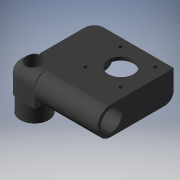
# Autodesk Inventor part: zmotormount
Saved by Autodesk Inventor 2019.1 (Build 231200000, 200)
## iProperties
Created: 2019-08-11
Part Number: zmotormount
Material: Generic
Document SubType Name: Modeling
Designer: rob
Density: 1 g/cm^3
Appearance: Default
Author: rob
## iProperties of the stored document zmotormount_3DPrint.ipt
Created: 2019-08-11
Part Number: zmotormount_3DPrint
Material: Generic
Document SubType Name: Modeling
Designer: rob
Density: 1 g/cm^3
Appearance: Default
Author: rob
Autodesk Inventor part; units mm, degrees
ref_plane "YZ Plane" through (0, 0, 0) normal (1, 0, 0) x (0, 1, 0)
ref_plane "XZ Plane" through (0, 0, 0) normal (0, 1, 0) x (-1, 0, 0)
ref_plane "XY Plane" through (0, 0, 0) normal (0, 0, 1) x (1, 0, 0)
sketch "Sketch1" plane through (0, 0, 0) normal (0, 1, 0) x (-1, 0, 0)
  circle A0 centre (0, 0) radius 9.125
  circle A1 centre (0, 0) radius 12.5
  dimension "d0" = 18.25
  dimension "d1" = 25
  constraints: 2 centre point, 2 coincident
  measures "d0" diameter of A0
  measures "d1" diameter of A1
extrude "Extrusion1" add sketch "Sketch1" along normal blind 15
sketch "Sketch2" plane through (0, 15, 0) normal (0, 1, 0) x (1, 0, 0)
  line L0 (-12.5, -12.5) -> (12.5, -12.5)
  line L1 (12.5, -12.5) -> (12.5, 12.5)
  line L2 (12.5, 12.5) -> (-12.5, 12.5)
  line L3 (-12.5, 12.5) -> (-12.5, -12.5)
  point P0 (0, 0)
  constraints: 8 end point, 2 parallel, 1 horizontal, 1 perpendicular
extrude "Extrusion2" add sketch "Sketch2" along normal blind 25
sketch "Sketch3" plane through (12.5, 15, 12.5) normal (1, 0, 0) x (0, 0, -1)
  circle A0 centre (12.5, 12.5) radius 12.5
  circle A1 centre (12.5, 12.5) radius 9.125
  point P0 (12.5, -15)
  dimension "d6" = 25
  dimension "d7" = 18.25
  constraints: 2 centre point, 1 coincident
  measures "d6" diameter of A0
  measures "d7" diameter of A1
extrude "Extrusion3" add sketch "Sketch3" along normal blind 53.5
fillet "Fillet1" radius 10 5 edges at (0, 40, -12.5) (-12.5, 40, 0) (0, 40, 12.5) (-12.5, 27.5, 12.5) (-12.5, 27.5, -12.5)
sketch "Sketch4" plane through (0, 40, 0) normal (0, 1, 0) x (1, 0, 0)
  circle A0 centre (43.7484, 32.8534) radius 11.25
  circle A1 centre (43.7484, 32.8534) radius 2.75
  circle A2 centre (28.2484, 17.3534) radius 1.75
  circle A3 centre (28.2484, 48.3534) radius 1.75
  circle A4 centre (59.2484, 48.3534) radius 1.75
  circle A5 centre (59.2484, 17.3534) radius 1.75
  line L0 (-2.5, -2.5) -> (-2.5, 2.5) projected
  line L1 (-2.5, -2.5) -> (55.5607, -2.5)
  line L2 (66, -2.5) -> (66, 83.8642)
  line L3 (55.5607, 83.8642) -> (-2.5, 83.8642)
  line L4 (-2.5, 83.8642) -> (-2.5, -2.5)
  line L5 (-47.4497, 33) -> (137.0981, 33)
  line L6 (43.6, -25.832) -> (43.6, 75.2549)
  line L7 (55.5607, 83.8642) -> (66, 83.8642)
  line L8 (66, -2.5) -> (47.9455, -2.5)
  line L9 (66, -12.5) -> (66, 12.5) projected
  point P0 (0, 0)
  dimension "d13" = 22.5
  dimension "d14" = 5.5
  dimension "d15" = 3.5
  dimension "d16" = 15.5
  dimension "d20" = 360
  dimension "d37" = 33
  dimension "d43" = 43.6
  dimension "d44" = 0
  constraints: 16 end point, 6 centre point, 3 coincident, 3 horizontal, 2 parallel, 1 perpendicular, 1 point on line, 1 vertical, 10 other
  measures "d13" diameter of A0
  measures "d14" diameter of A1
  measures "d15" diameter of A2
  measures "d16" horizontal distance of A2.centre A0.centre
  measures "d37" distance from line of L5 point (0, 0)
  measures "d43" distance from line of L6 point (0, 0)
  measures "d44" distance between parallel lines of L9 L2
extrude "Extrusion4" add sketch "Sketch4" against normal blind 3 contours A0 L5 L2 L8 L1 L6 | A0 L5 L4 L3 L7 L2 | L6 L1 L0 L4 L5 A0
fillet "Fillet2" radius 40 1 edges at (-2.5, 38.5, -83.8642)
fillet "Fillet3" radius 10 1 edges at (66, 38.5, -83.8642)
sketch "Sketch5" plane through (66, 27.5, 0) normal (1, 0, 0) x (0, 0, -1)
  circle A0 centre (0, 0) radius 12.5
  line L0 (0, -12.5) -> (-12.5, -12.5) projected
  line L1 (0, -12.5) -> (73.8642, -12.5)
  line L2 (83.8642, 9.5) -> (83.8642, 12.5) projected
  line L3 (73.8642, -12.5) -> (73.8642, 12.5)
  line L4 (73.8642, 12.5) -> (0, 12.5)
  circle A1 centre (0, 0) radius 9.125
  line L5 (73.8642, 12.5) -> (73.8642, 9.5) projected
  point P0 (0, -27.5)
  dimension "d28" = 0
  dimension "d45" = 18.25
  constraints: 5 end point, 2 centre point, 2 tangent, 1 coincident, 1 collinear, 1 perpendicular, 1 point on circle, 1 point on line
  measures "d28" distance between parallel lines of L5 L3
  measures "d45" diameter of A1
extrude "Extrusion5" add sketch "Sketch5" along normal blind 2
fillet "Fillet5" radius 8 2 edges at (67, 15, -73.8642) (68, 27.5, -73.8642)
sketch "Sketch6" plane through (12.5, 15, 0) normal (1, 0, 0) x (0, 0, -1)
  line L0 (12.5, 15) -> (12.5, 0) projected
  line L1 (12.5, 0) -> (65.8642, 0)
  line L2 (0, 0) -> (65.8642, 0) projected
  line L3 (65.8642, 0) -> (65.8642, 22)
  line L4 (44.1034, 22) -> (21.6034, 22) projected
  line L5 (65.8642, 0) -> (12.5, 0)
  line L6 (12.5, 0) -> (12.5, 22)
  line L7 (12.5, 22) -> (65.8642, 22)
  line L8 (65.8642, 22) -> (65.8642, 0)
  point P0 (0, -15)
  point P1 (12.5, 14.9361)
  constraints: 12 end point, 2 horizontal, 2 parallel, 2 point on line, 1 perpendicular, 1 vertical
extrude "Extrusion6" add sketch "Sketch6" along normal blind 2
fillet "Fillet6" radius 8 1 edges at (13.5, 15, -65.8642)
sketch "Sketch7" plane through (0, 0, 0) normal (0, -1, 0) x (1, 0, 0)
  circle A0 centre (0, 0) radius 8.975
  constraints: 1 centre point, 1 coincident
extrude "Extrusion7" cut sketch "Sketch7" against normal blind 25
sketch "Sketch8" plane through (0, 37, 0) normal (0, -1, 0) x (1, 0, 0)
  line L0 (-23.3822, -55.3999) -> (103.7661, -55.3999)
  line L1 (103.7661, -55.3999) -> (103.7661, -98.1886)
  line L2 (103.7661, -98.1886) -> (-23.3822, -98.1886)
  line L3 (-23.3822, -98.1886) -> (-23.3822, -55.3999)
  point P0 (0, 0)
  constraints: 8 end point, 2 parallel, 1 horizontal, 1 perpendicular
extrude "Extrusion8" cut sketch "Sketch8" along normal mid plane 200
fillet "Fillet7" radius 8 3 edges at (-0.8005, 38.5, -55.3999) (13.5, 15, -55.3999) (67, 15, -55.3999)
extrude "Extrusion9" cut sketch "Sketch4" against normal blind 200 contours A2 | A5
sketch "Sketch9" plane through (0, 25, 0) normal (0, -1, 0) x (1, 0, 0)
  circle A0 centre (0, 0) radius 7.5
  dimension "d46" = 15
  constraints: 1 centre point, 1 coincident
  measures "d46" diameter of A0
extrude "Extrusion10" cut sketch "Sketch9" against normal blind 60
body "Solid1"
